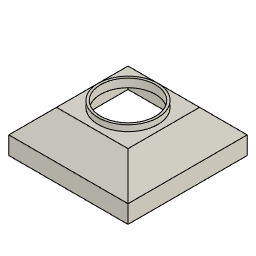
Joystick Assembly v10 (Autodesk Fusion 360 archive; units mm, degrees)
design "Base"
Autodesk Fusion 360 part; units mm, degrees
sketch "Sketch1" plane through (0, 0, 0) normal (0, 0, 1) x (1, 0, 0)
  line L0 (-50, 50) -> (50, 50)
  line L1 (50, 50) -> (50, -50)
  line L2 (50, -50) -> (-50, -50)
  line L3 (-50, -50) -> (-50, 50)
  constraint horizontal L0
  constraint vertical L1
  constraint horizontal L2
  constraint vertical L3
extrude "Extrude1" add sketch "Sketch1" along normal blind 35
chamfer "Chamfer1" distance 20 angle 45 4 edges at (50, 0, 35) (0, -50, 35) (-50, 0, 35) (0, 50, 35)
sketch "Sketch2" plane through (0, 0, 35) normal (0, 0, 1) x (-1, 0, 0)
  line L0 (30, -30) -> (30, 30)
  line L1 (30, 30) -> (-30, 30)
  line L2 (-30, 30) -> (-30, -30)
  line L3 (-30, -30) -> (30, -30)
  circle A0 centre (0, 0) radius 25
  constraint coincident A0.centre origin
extrude "Extrude2" add sketch "Sketch2" along normal blind 5 contours A0
shell "Shell1" thickness 2 removed faces 2 at (-16.6667, 16.6667, 0) at (6.7759, 1.242, 40)

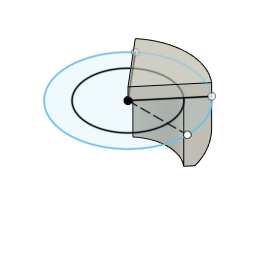
design "trigger"
Autodesk Fusion 360 part; units mm, degrees
sketch "Sketch1" plane through (0, 0, 0) normal (0, 0, 1) x (1, 0, 0)
  circle A0 centre (0, 0) radius 15
  line L0 (0, 0) -> (-9.6418, 11.4907)
  line L1 (0, 0) -> (15, 0) construction
  line L2 (0, 0) -> (9.6418, 11.4907)
  line L3 (0, 0) -> (15, 0) construction
  circle A1 centre (0, 0) radius 10
  dimension "d1" = 130
  dimension "d2" = 50
  dimension "d3" = 20
  constraint coincident A0.centre L0.start
  constraint horizontal L1
  constraint horizontal L3
  measures "d1" angle of L0 L1
  measures "d2" angle of L2 L3
  measures "d3" diameter of A1
extrude "Extrude1" add sketch "Sketch1" along normal blind 3 contours A0 L0 L2 A1 | L0 L2 A1 picked at (-7.6299, 10.8973) picked at (-2.2746, 6.2494)
extrude "Extrude2" add sketch "Sketch1" against normal blind 15 contours A0 L0 L2 A1 picked at (-7.6299, 10.8973)
chamfer "Chamfer1" distance 3 angle 45 1 edges at (0, 15, -15)
fillet "Fillet1" radius 12 1 edges at (0, 15, -12)

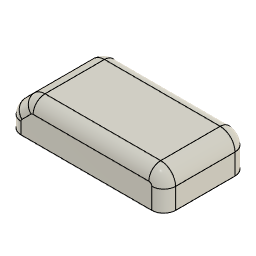
design "Bumper"
Autodesk Fusion 360 part; units mm, degrees
sketch "Sketch1" plane through (0, 0, 0) normal (0, 0, 1) x (1, 0, 0)
  line L0 (-10, 5) -> (16, 5)
  line L1 (16, 5) -> (16, -9)
  line L2 (16, -9) -> (-10, -9)
  line L3 (-10, -9) -> (-10, 5)
  constraint horizontal L0
  constraint vertical L1
  constraint horizontal L2
  constraint vertical L3
extrude "Extrude1" add sketch "Sketch1" along normal blind 6
chamfer "Chamfer1" distance 3 angle 45 1 edges at (-10, -2, 6)
fillet "Fillet1" radius 2.5 3 edges at (-7, -2, 6) (-10, -2, 3) (16, -2, 6)
fillet "Fillet2" radius 2 14 edges at (-10, -9, 0.9822) (-9.8097, -9, 2.9212) (-8.5, -9, 4.5) (-6.9212, -9, 5.8097) (3.7678, -9, 6) (15.2678, -9, 5.2678) (16, -9, 1.75) (16, 5, 1.75) (15.2678, 5, 5.2678) (3.7678, 5, 6) (-6.9212, 5, 5.8097) (-8.5, 5, 4.5) (-9.8097, 5, 2.9212) (-10, 5, 0.9822)

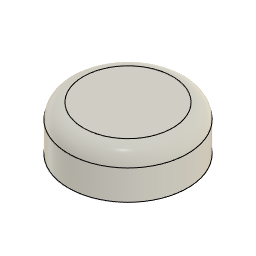
design "Start Button"
Autodesk Fusion 360 part; units mm, degrees
sketch "Sketch1" plane through (0, 0, 0) normal (0, 0, 1) x (1, 0, 0)
  circle A0 centre (0, 0) radius 4
  dimension "d1" = 8
  constraint coincident A0.centre origin
  measures "d1" diameter of A0
extrude "Extrude1" add sketch "Sketch1" along normal blind 3
fillet "Fillet1" radius 1 1 edges at (-3.7293, -1.4465, 3)

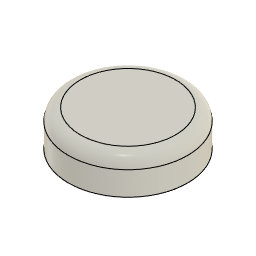
design "Face Button"
Autodesk Fusion 360 part; units mm, degrees
sketch "Sketch1" plane through (0, 0, 0) normal (0, 0, 1) x (1, 0, 0)
  circle A0 centre (0, 0) radius 5
  dimension "d1" = 10
  constraint coincident A0.centre origin
  measures "d1" diameter of A0
extrude "Extrude1" add sketch "Sketch1" along normal blind 3
fillet "Fillet1" radius 1 1 edges at (-4.6616, -1.8081, 3)

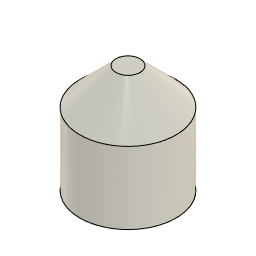
design "Hat"
Autodesk Fusion 360 part; units mm, degrees
sketch "Sketch1" plane through (0, 0, 0) normal (0, 0, 1) x (1, 0, 0)
  circle A0 centre (0, 0) radius 8
  dimension "d1" = 16
  constraint coincident A0.centre origin
  measures "d1" diameter of A0
extrude "Extrude1" add sketch "Sketch1" along normal blind 18
chamfer "Chamfer1" distance 6 angle 45 1 edges at (-7.4586, -2.8929, 18)
